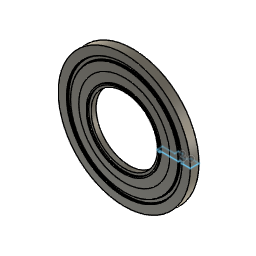
Design A Spacer (Autodesk Fusion 360 design; units mm, degrees)
Autodesk Fusion 360 part; units mm, degrees
note: some values were not read from the file. Set by a fixed rule: which sketch regions a step uses.
sketch "Sketch1" plane through (0, 0, 0) normal (0, 0, 1) x (1, 0, 0)
  spline S0 degree 5 poles (40.3, 8.0005) (40.3854, 8.0005) (40.5575, 7.9418) (40.8197, 7.6776) (41.2001, 7.0315) (41.8406, 6.0459) (42.7193, 5.2457) (43.8506, 4.9398) (44.9792, 5.2641) (45.8516, 6.0676) (46.4866, 7.0454) (46.8672, 7.6822) (47.134, 7.9422) (47.3114, 8) (47.4, 8) knots 0 0 0 0 0 0 0.1 0.2 0.3 0.4 0.5 0.6 0.7 0.8 0.9 1 1 1 1 1 1
  line L0 (40.3, 8.0005) -> (36.9987, 8.0005)
  line L1 (47.4, 8) -> (53.6987, 8)
  line L2 (47.1403, 8) -> (47.6598, 8)
  line L3 (40.0497, 8.0005) -> (40.5503, 8.0005)
  line L4 (53.6987, 8) -> (53.6987, 1.0001)
  line L5 (43.2, 5.0899) -> (44.5, 5.1)
  line L6 (46.7394, 0.9997) -> (46.7394, 2.3197)
  line L7 (46.7394, 2.3197) -> (43.9694, 2.3205)
  line L8 (43.9694, 2.3205) -> (43.9694, 1.0001)
  line L9 (37, 1) -> (43.9694, 1.0001)
  line L10 (46.7394, 0.9997) -> (53.6987, 1.0001)
  line L11 (36.9987, 8.0005) -> (37.0139, 5.0519)
  line L12 (37.0139, 5.0519) -> (26.9987, 5.0003)
  line L13 (26.9987, 5.0003) -> (26.9987, 1)
  line L14 (26.9987, 1) -> (28.9987, 1)
  line L15 (28.9987, 1) -> (28.9987, 0)
  line L16 (28.9987, 0) -> (29.9987, 0)
  line L17 (29.9987, 0) -> (29.9987, 1)
  line L18 (29.9987, 1) -> (37, 1)
  point P0 (43.85, 5.095)
  dimension "d4" = 16.7
  dimension "d19" = 1.32
  dimension "d20" = 2.77
  dimension "d30" = 2
  dimension "d31" = 1
  dimension "d32" = 1
  constraint parallel L0 L1
  constraint midpoint L2 S0.end
  constraint coincident L1 L2.end
  constraint midpoint L3 S0.start
  constraint coincident L0 L3.start
  constraint midpoint P0 L5
  constraint coincident L1 S0.end
  constraint coincident L0 S0.start
  constraint perpendicular L13 L14
  constraint perpendicular L14 L15
  constraint perpendicular L15 L16
  measures "d4" distance of L1.end L0.end
  measures "d19" distance of L6.start L6.end
  measures "d20" distance of L6.end L7.end
  measures "d30" distance of L13.end L14.end
  measures "d31" distance of L14.end L15.end
  measures "d32" distance of L15.end L16.end
revolve "Revolve1" add sketch "Sketch1" angle 360 about axis through (0, 1.75, 0) along (0, 1, 0)
fillet "Fillet1" radius 0.25 1 edges at (-40.9938, 2.3205, -15.9)
fillet "Fillet2" radius 0.25 1 edges at (-43.5764, 2.3197, -16.9017)
fillet "Fillet3" radius 0.25 1 edges at (-40.9938, 1.0001, -15.9)
fillet "Fillet4" radius 0.25 1 edges at (-43.5764, 0.9997, -16.9017)
